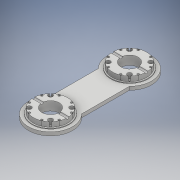
# Autodesk Inventor part: tri_fore_arm_step_6810
Saved by Autodesk Inventor 2017 (Build 210142000, 142)
## iProperties
Created: 2019-06-14
Part Number: tri_fore_arm_step_6810
Material: Generic
Document SubType Name: Modeling
Designer: paulg
Density: 1 g/cm^3
Appearance: Default
Author: paulg
Autodesk Inventor part; units mm, degrees
ref_plane "YZ Plane" through (0, 0, 0) normal (1, 0, 0) x (0, 1, 0)
ref_plane "XZ Plane" through (0, 0, 0) normal (0, 1, 0) x (-1, 0, 0)
sketch "Sketch1" plane through (0, 0, 0) normal (0, 0, 1) x (1, 0, 0)
  circle A0 centre (0, 0) radius 25
  circle A1 centre (0, 0) radius 5
  dimension "d0" = 50
  dimension "d1" = 10
  constraints: 2 centre point, 2 coincident
  measures "d0" diameter of A0
  measures "d1" diameter of A1
extrude "Extrusion1" add sketch "Sketch1" along normal blind 7
sketch "Sketch2" plane through (0, 0, 0) normal (0, 0, -1) x (-1, 0, 0)
  circle A0 centre (0, 0) radius 5 projected
  circle A1 centre (0, 0) radius 25 projected
  circle A2 centre (0, 0) radius 27
  dimension "d4" = 2
  constraints: 1 centre point, 1 coincident
  measures "d4" radial gap between concentric circles of A1 A2
extrude "Extrusion2" add sketch "Sketch2" along normal blind 1 contours A1 | A2
sketch "Sketch3" plane through (0, 0, -1) normal (0, 0, -1) x (-1, 0, 0)
  circle A0 centre (0, 0) radius 5 projected
  circle A1 centre (0, 0) radius 27 projected
  circle A2 centre (0, 0) radius 32
  dimension "d7" = 64
  constraints: 1 centre point, 1 coincident
  measures "d7" diameter of A2
extrude "Extrusion3" add sketch "Sketch3" along normal blind 5 contours A1 | A2
sketch "Sketch4" plane through (0, 0, 7) normal (0, 0, 1) x (1, 0, 0)
  circle A0 centre (0, 0) radius 5
  circle A1 centre (0, 0) radius 25
  line L0 (0, 0) -> (23.096988, 9.567086) construction
  circle A2 centre (21.711169, 8.993061) radius 1.5
  circle A3 centre (8.993061, 21.711169) radius 1.5
  circle A4 centre (-8.993061, 21.711169) radius 1.5
  circle A5 centre (-21.711169, 8.993061) radius 1.5
  circle A6 centre (-21.711169, -8.993061) radius 1.5
  circle A7 centre (-8.993061, -21.711169) radius 1.5
  circle A8 centre (8.993061, -21.711169) radius 1.5
  circle A9 centre (0, 0) radius 25
  line L1 (0, 0) -> (25, 0) construction
  circle A10 centre (21.711169, -8.993061) radius 1.5
  line L2 (0, 0) -> (21.711169, -8.993061) construction
  point P0 (9.567086, 23.096988)
  point P1 (-9.567086, 23.096988)
  point P2 (-23.096988, 9.567086)
  point P3 (-23.096988, -9.567086)
  point P4 (-9.567086, -23.096988)
  point P5 (9.567086, -23.096988)
  point P6 (23.096988, -9.567086)
  dimension "d10" = 3
  dimension "d13" = 360
  constraints: 6 end point, 4 point on circle, 1 horizontal, 1 point on line, 51 other
extrude "Extrusion4" cut sketch "Sketch4" against normal blind 6 contours A2 | A4 | A6 | A8 | A10 | A7 | A5 | A3
sketch "Sketch5" plane through (0, 0, -6) normal (0, 0, -1) x (-1, 0, 0)
  circle A0 centre (0, 0) radius 5 projected
  circle A1 centre (0, 0) radius 32 projected
  circle A2 centre (0, 0) radius 12.5
  dimension "d17" = 25
  constraints: 1 centre point, 1 coincident
  measures "d17" diameter of A2
extrude "Extrusion5" cut sketch "Sketch5" against normal through all contours A2
sketch "Sketch6" plane through (0, 0, -6) normal (0, 0, -1) x (-1, 0, 0)
  circle A0 centre (0, 0) radius 12.5
  circle A1 centre (0, 0) radius 32
  line L0 (13.711309, -21.5) -> (-13.711309, -21.5)
  line L1 (-21.5, -13.711309) -> (-21.5, 13.711309)
  line L2 (-13.711309, 21.5) -> (13.711309, 21.5)
  line L3 (21.5, 13.711309) -> (21.5, -13.711309)
  line L4 (21.5, -21.5) -> (-21.5, 21.5) construction
  line L5 (-21.5, -21.5) -> (21.5, 21.5) construction
  arc A2 (21.5, 13.711309) -> (13.711309, 21.5) centre (0, 0) ccw
  arc A3 (13.711309, -21.5) -> (21.5, -13.711309) centre (0, 0) ccw
  arc A4 (-13.711309, 21.5) -> (-21.5, 13.711309) centre (0, 0) ccw
  arc A5 (-21.5, -13.711309) -> (-13.711309, -21.5) centre (0, 0) ccw
  line L6 (0, 0) -> (32, 0) construction
  line L7 (0, 0) -> (0, -32) construction
  dimension "d20" = 43
  dimension "d22" = 25.5
  dimension "d23" = 43
  dimension "d24" = 43
  constraints: 16 end point, 10 point on circle, 4 centre point, 3 concentric, 2 horizontal, 2 midpoint, 2 parallel, 1 coincident, 1 perpendicular, 1 vertical, 2 other
  measures "d20" distance of L4.end L5.end
  measures "d22" radius of A2
  measures "d23" distance between parallel lines of L0 L2
  measures "d24" distance between parallel lines of L3 L1
extrude "Extrusion6" [suppressed]
sketch "Sketch7" plane through (0, 0, -1) normal (0, 0, 1) x (1, 0, 0)
  circle A0 centre (-21.711169, -8.993061) radius 1.5
  circle A1 centre (-8.993061, -21.711169) radius 1.5
  line L0 (15.5, -15.5) -> (-15.5, -15.5) construction
  line L1 (-15.5, -15.5) -> (-15.5, 15.5) construction
  line L2 (-15.5, 15.5) -> (15.5, 15.5) construction
  line L3 (15.5, 15.5) -> (15.5, -15.5) construction
  line L4 (15.5, -15.5) -> (-15.5, 15.5) construction
  line L5 (-15.5, -15.5) -> (15.5, 15.5) construction
  point P0 (0, 0)
  point P1 (-23.096988, -9.567086)
  point P2 (-9.567086, -23.096988)
  dimension "d76" = 31
  constraints: 12 end point, 4 coincident, 2 midpoint, 2 parallel, 2 perpendicular, 1 horizontal, 2 other
  measures "d76" distance of L0.start L0.end
hole "Hole1" at (15.5, 15.5, -1) at (-15.5, 15.5, -1) at (-15.5, -15.5, -1) at (15.5, -15.5, -1) direction (0, 0, 1) diameter 6.5 end through all
ref_plane "Work Plane1" through (-18.444138, -16.876426, 90.438504) normal (0, 1, 0) x (0, 0, 1)
sketch "Sketch9" plane through (0, 0, -6) normal (0, 0, -1) x (-1, 0, 0)
  line L0 (0, 0) -> (0, -32) construction
  circle A0 centre (0, 0) radius 32
  line L1 (0, 0) -> (0, -32) construction
  line L2 (-22.5, -22.754121) -> (22.5, -22.754121) construction
  line L3 (22.5, -22.754121) -> (22.5, -57.5)
  line L4 (22.5, -57.5) -> (-22.5, -57.5)
  line L5 (-22.5, -57.5) -> (-22.5, -22.754121)
  line L6 (-22.5, -22.754121) -> (22.5, -57.5) construction
  line L7 (22.5, -22.754121) -> (-22.5, -57.5) construction
  circle A1 centre (0, 0) radius 32
  arc A2 (-22.5, -22.754121) -> (22.5, -22.754121) centre (0, 0) ccw
  point P0 (0, -40.12706)
  dimension "d40" = 0
  dimension "d41" = 45
  dimension "d45" = 57.5
  constraints: 16 end point, 5 point on circle, 3 point on line, 2 midpoint, 2 perpendicular, 1 centre point, 1 parallel, 1 vertical, 3 other
  measures "d40" distance between parallel lines of L1 L0
  measures "d41" distance of L3.end L4.end
  measures "d45" distance from line of L4 L0.start
extrude "Extrusion8" add sketch "Sketch9" against normal up to surface (5 mm away) contours A0 L3 L4 L5
sketch "Sketch10" plane through (0, 0, -6) normal (0, 0, -1) x (-1, 0, 0)
  circle A0 centre (0, 0) radius 12.5
  arc A1 (22.5, -22.754121) -> (-22.5, -22.754121) centre (0, 0) ccw
  line L0 (-22.5, -22.754121) -> (-22.5, -57.5)
  line L1 (-22.5, -57.5) -> (22.5, -57.5)
  line L2 (22.5, -57.5) -> (22.5, -22.754121)
  line L3 (0, 0) -> (0, -57.5) construction
  line L4 (-22.5, -57.5) -> (22.5, -57.5) construction
  line L5 (-15, 53.5) -> (-15, -53.5) construction
  line L6 (-15, -53.5) -> (15, -53.5) construction
  line L7 (15, -53.5) -> (15, 53.5) construction
  line L8 (15, 53.5) -> (-15, 53.5) construction
  line L9 (-15, 53.5) -> (15, -53.5) construction
  line L10 (-15, -53.5) -> (15, 53.5) construction
  line L11 (33, 41.5) -> (33, -41.5) construction
  line L12 (33, -41.5) -> (-33, -41.5) construction
  line L13 (-33, -41.5) -> (-33, 41.5) construction
  line L14 (-33, 41.5) -> (33, 41.5) construction
  line L15 (33, 41.5) -> (-33, -41.5) construction
  line L16 (33, -41.5) -> (-33, 41.5) construction
  line L17 (30, 53.5) -> (30, -53.5) construction
  line L18 (30, -53.5) -> (-30, -53.5) construction
  line L19 (-30, -53.5) -> (-30, 53.5) construction
  line L20 (-30, 53.5) -> (30, 53.5) construction
  line L21 (30, 53.5) -> (-30, -53.5) construction
  line L22 (30, -53.5) -> (-30, 53.5) construction
  dimension "d46" = 4
  dimension "d47" = 16
  dimension "d48" = 30
  dimension "d49" = 66
  dimension "d73" = 4
  dimension "d74" = 60
  constraints: 38 end point, 7 midpoint, 6 coincident, 6 parallel, 3 perpendicular
  measures "d46" distance between parallel lines of L1 L6
  measures "d47" distance between parallel lines of L1 L12
  measures "d48" distance of L5.end L6.end
  measures "d49" distance of L11.end L12.end
  measures "d73" distance between parallel lines of L18 L1
  measures "d74" distance of L17.end L18.end
hole "Hole2" [suppressed]
chamfer "Chamfer1" [suppressed]
sketch "Sketch11" plane through (0, 0, -1) normal (0, 0, 1) x (1, 0, 0)
  line L0 (22.5, -57.5) -> (-22.5, -57.5)
  line L1 (22.5, -22.754121) -> (22.5, -57.5)
  arc A0 (22.5, -22.754121) -> (-22.5, -22.754121) centre (0, 0) ccw
  line L2 (-22.5, -57.5) -> (-22.5, -22.754121)
  circle A1 centre (0, 0) radius 27
  circle A2 centre (-15.5, 15.5) radius 3.25
  circle A3 centre (15.5, 15.5) radius 3.25
  circle A4 centre (-15.5, -15.5) radius 3.25
  circle A5 centre (15.5, -15.5) radius 3.25
  constraints: 4 coincident
hole "Hole3" at (-15.5, -15.5, -1) at (-15.5, 15.5, -1) at (15.5, 15.5, -1) at (15.5, -15.5, -1) direction (0, 0, -1) diameter 3 end through all countersink diameter 6.5 countersink angle 90
sketch "Sketch12" plane through (0, 0, -6) normal (0, 0, -1) x (-1, 0, 0)
  circle A0 centre (21.711169, 8.993061) radius 1.5
  circle A1 centre (-21.664975, -8.973926) radius 1.55
  point P0 (0, 0)
  point P1 (-23.096988, -9.567086)
  point P2 (23.096988, 9.567086)
  constraints: 2 other
extrude "Extrusion9" cut sketch "Sketch12" against normal through all
sketch "Sketch13" plane through (0, 0, -6) normal (0, 0, -1) x (-1, 0, 0)
  circle A0 centre (-21.664975, -8.973926) radius 1.55
  circle A1 centre (-15.5, 15.5) radius 1.5
  circle A2 centre (15.5, -15.5) radius 1.5
  circle A3 centre (15.5, 15.5) radius 1.5
  circle A4 centre (-15.5, -15.5) radius 1.5
  circle A5 centre (0, 0) radius 12.5
  line L0 (22.5, -57.5) -> (22.5, -22.754121)
  arc A6 (22.5, -22.754121) -> (-22.5, -22.754121) centre (0, 0) ccw
  line L1 (-22.5, -22.754121) -> (-22.5, -57.5)
  line L2 (-22.5, -57.5) -> (22.5, -57.5)
  line L3 (22.057822, 11.626151) -> (24.164819, 10.009396)
  line L4 (24.164819, 10.009396) -> (23.818166, 7.376305)
  line L5 (23.818166, 7.376305) -> (21.364516, 6.35997)
  line L6 (21.364516, 6.35997) -> (19.257519, 7.976726)
  line L7 (19.257519, 7.976726) -> (19.604172, 10.609816)
  line L8 (19.604172, 10.609816) -> (22.057822, 11.626151)
  line L9 (-21.318322, -6.340836) -> (-19.211325, -7.957592)
  line L10 (-19.211325, -7.957592) -> (-19.557978, -10.590682)
  line L11 (-19.557978, -10.590682) -> (-22.011628, -11.607017)
  line L12 (-22.011628, -11.607017) -> (-24.118625, -9.990261)
  line L13 (-24.118625, -9.990261) -> (-23.771972, -7.357171)
  line L14 (-23.771972, -7.357171) -> (-21.318322, -6.340836)
  circle A7 centre (21.711169, 8.993061) radius 1.5
  line L15 (21.711169, 8.993061) -> (-21.664975, -8.973926) construction
  dimension "d69" = 4.6
  dimension "d70" = 4.6
  constraints: 26 end point, 2 coincident, 2 parallel, 26 other
  measures "d69" distance between parallel lines of L5 L8
  measures "d70" distance between parallel lines of L11 L14
extrude "Extrusion10" cut sketch "Sketch13" against normal blind 3.5 contours A0 | L3 L4 L5 L6 L7 L8 | L9 L10 L11 L12 L13 L14 | A7
sketch "Sketch14" plane through (0, 0, 0) normal (1, 0, 0) x (0, 1, 0)
  line L0 (9.567086, 7) -> (9.567086, 0)
  line L1 (-16.876426, 0) -> (9.567086, 0)
  line L2 (-16.876426, 0) -> (-16.876426, 7)
  line L3 (-9.567086, 7) -> (-16.876426, 7)
  line L4 (16.876426, 7) -> (9.567086, 7)
  line L5 (16.876426, 7) -> (16.876426, 0)
  circle A0 centre (0, 7) radius 2
  line L6 (16.876426, 0) -> (16.876426, 7)
  line L7 (18.444138, 7) -> (18.444138, 0)
  line L8 (18.444138, 0) -> (18.444138, 0)
  line L9 (18.444138, 0) -> (18.444138, 7)
  line L10 (-18.444138, 7) -> (-18.444138, 0)
  line L11 (-18.444138, 0) -> (-18.444138, 0)
  line L12 (-18.444138, 0) -> (-18.444138, 7)
  line L13 (-16.876426, 7) -> (-16.876426, 0)
  line L14 (9.567086, 7) -> (16.876426, 7)
  line L15 (9.567086, 7) -> (9.567086, 1)
  line L16 (23.096988, 7) -> (18.444138, 7)
  line L17 (23.096988, 7) -> (23.096988, 1)
  line L18 (23.096988, 7) -> (23.096988, 7)
  line L19 (23.096988, 7) -> (23.096988, 1)
  line L20 (-23.096988, 7) -> (-23.096988, 1)
  line L21 (-9.567086, 7) -> (-9.567086, 1)
  line L22 (-23.096988, 7) -> (-23.096988, 1)
  line L23 (-9.567086, 7) -> (9.567086, 7)
  line L24 (16.876426, 0) -> (-9.567086, 0)
  line L25 (18.444138, 7) -> (23.096988, 7)
  line L26 (-23.096988, 7) -> (-23.096988, 7)
  line L27 (-18.444138, 7) -> (-23.096988, 7)
  line L28 (-9.567086, 7) -> (-9.567086, 0)
  line L29 (-16.876426, 7) -> (-9.567086, 7)
  line L30 (-23.096988, 7) -> (-18.444138, 7)
  line L31 (-9.567086, 0) -> (-16.876426, 0)
  line L32 (9.567086, 0) -> (16.876426, 0)
  line L33 (9.567086, 7) -> (-9.567086, 7)
  point P0 (0, 0)
  dimension "d77" = 4
  constraints: 1 centre point
  measures "d77" diameter of A0
extrude "Extrusion11" cut sketch "Sketch14" along normal through all both and the other way through all contours L23 A0 | A0 L23
mirror "Mirror1" about plane through (-22.5, -57.5, -6) normal (0, -1, 0) of "Extrusion1", "Extrusion2", "Extrusion3", "Extrusion4", "Extrusion5", "Hole1", "Extrusion8", "Hole3", "Extrusion9", "Extrusion10", "Extrusion11"
ref_plane "Work Plane2" through (-18.444138, -98.123574, 90.438504) normal (0, 1, 0) x (0, 0, 1)
equation "\"d24\" = d23"
equation "\"d70\" = d69"
body "Solid1"
